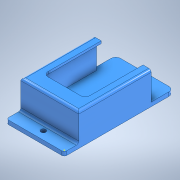
# Autodesk Inventor part: Camera_Mount
Saved by Autodesk Inventor 2022 (Build 260153000, 153)
## iProperties
Created: 2021-06-15
Part Number: Camera_Mount
Material: Generic
Document SubType Name: Modeling
Designer: Jorian Brusind
Density: 1 g/cm^3
Appearance: Cyan
Author: Jorian Brusind
Autodesk Inventor part; units mm, degrees
ref_plane "YZ Plane" through (0, 0, 0) normal (1, 0, 0) x (0, 1, 0)
ref_plane "XZ Plane" through (0, 0, 0) normal (0, 1, 0) x (-1, 0, 0)
ref_plane "XY Plane" through (0, 0, 0) normal (0, 0, 1) x (1, 0, 0)
sketch "Sketch1" plane through (0, 0, 0) normal (0, 1, 0) x (-1, 0, 0)
  line L0 (0, 0) -> (68, 0)
  line L1 (68, 0) -> (68, -132)
  line L2 (68, -132) -> (0, -132)
  line L3 (0, -132) -> (0, 0)
  line L4 (70, -134) -> (70, 2)
  line L5 (70, 2) -> (-2, 2)
  line L6 (-2, 2) -> (-2, -134)
  line L7 (-2, -134) -> (70, -134)
  dimension "d0" = 68
  dimension "d1" = 132
  dimension "d2" = 2
  constraints: 16 end point, 4 parallel, 2 perpendicular, 1 horizontal, 3 other
  measures "d0" distance of L1.end L2.end
  measures "d1" distance of L0.end L1.end
  measures "d2" distance between parallel lines of L1 L4
extrude "Extrusion1" add sketch "Sketch1" along normal blind 3 contours L0 L1 L2 L3 | L7 L6 L5 L4
sketch "Sketch2" plane through (0, 3, 0) normal (0, 1, 0) x (1, 0, 0)
  line L0 (2, 134) -> (-70, 134) projected
  line L1 (-70, -2) -> (2, -2) projected
  line L2 (-70, 134) -> (2, 134)
  line L3 (2, 134) -> (2, -2)
  line L4 (2, -2) -> (-70, -2)
  line L5 (-70, -2) -> (-70, 134)
  line L6 (-70, 134) -> (-70, -2) projected
  line L7 (-70, 66) -> (2, 66)
  line L8 (2, -2) -> (2, 134) projected
  line L9 (-2, 106) -> (-66, 106)
  line L10 (-66, 106) -> (-66, 20)
  line L11 (-66, 20) -> (-2, 20)
  line L12 (-2, 20) -> (-2, 106)
  line L13 (2, 110) -> (-70, 110)
  line L14 (-70, 110) -> (-70, 16)
  line L15 (-70, 16) -> (2, 16)
  line L16 (2, 16) -> (2, 110)
  line L17 (-66, 106) -> (-70, 106)
  line L18 (-2, 106) -> (2, 106)
  point P0 (0, 0)
  point P1 (-70, -2)
  point P2 (-34, 66)
  point P3 (-30, 72)
  point P4 (-70, 106)
  point P5 (-70, 16)
  point P6 (2, 16)
  point P7 (2, 106)
  dimension "d113" = 64
  dimension "d114" = 86
  dimension "d115" = 72
  dimension "d116" = 94
  dimension "d149" = 40
  dimension "d150" = 44
  dimension "d180" = 32
  dimension "d181" = 36
  constraints: 30 end point, 6 parallel, 4 perpendicular, 3 horizontal, 3 midpoint, 3 point on line
  measures "d113" distance of L11.end L10.end
  measures "d114" distance of L10.end L9.end
  measures "d115" distance of L15.end L14.end
  measures "d116" distance of L14.end L13.end
  measures "d149" distance between parallel lines of L9 L7
  measures "d150" distance between parallel lines of L13 L7
  measures "d180" distance from line of point (-34, 66) L10
  measures "d181" distance from line of L14 point (-34, 66)
extrude "Extrusion2" add sketch "Sketch2" along normal blind 32 contours L3 L7 L12 L18 | L17 L10 L7 L5 | L3 L15 L5 L7 L10 L11 L12
sketch "Sketch3" plane through (0, 0, 0) normal (0, -1, 0) x (1, 0, 0)
  circle A0 centre (-34, -96) radius 2
  circle A1 centre (-34, -36) radius 2
  circle A2 centre (-51.5, -66) radius 2
  circle A3 centre (-16.5, -66) radius 2
  line L0 (2, -134) -> (-70, -134) projected
  line L1 (-70, -134) -> (-70, 2) projected
  line L2 (-70, -66) -> (2, -66)
  line L3 (2, 2) -> (2, -134) projected
  point P0 (0, 0)
  dimension "d10" = 4
  dimension "d13" = 60
  dimension "d14" = 35
  dimension "d15" = 17.5
  dimension "d16" = 30
  dimension "d17" = 30
  dimension "d18" = 17.5
  dimension "d117" = 30
  dimension "d202" = 36
  constraints: 4 centre point, 3 equal radius, 2 end point, 2 midpoint
  measures "d10" diameter of A1
  measures "d13" distance of A1.centre A0.centre
  measures "d14" distance of A3.centre A2.centre
  measures "d15" horizontal distance of A2.centre A0.centre
  measures "d16" vertical distance of A3.centre A0.centre
  measures "d17" vertical distance of A0.centre A2.centre
  measures "d18" horizontal distance of A1.centre A3.centre
  measures "d117" distance from line of L2 A0.centre
  measures "d202" distance from line of L1 A0.centre
extrude "Extrusion3" cut sketch "Sketch3" against normal through all contours A0 | A1 | L2 A2 | A2 L2 | L2 A3 | A3 L2
ref_plane "Work Plane3" through (-62, 3, 10) normal (0, 1, 0) x (1, 0, 0)
ref_plane "Work Plane4" through (-62, 30, 10) normal (0, 1, 0) x (1, 0, 0)
move faces "Move2" translate (0, -2, 0) faces at (-34.0804, 0, -10.0049)
fillet "Fillet17" radius 6 2 edges at (-70, 0.5, -134) (2, 0.5, -134)
ref_plane "Work Plane5" through (-9, -2, 2) normal (0, -1, 0) x (1, 0, 0)
ref_plane "Work Plane7" through (-62, 35, 10) normal (0, 1, 0) x (1, 0, 0)
ref_plane "Work Plane6" through (-62, 35, 10) normal (0, 1, 0) x (1, 0, 0)
sketch "Sketch16" plane through (0, 3, 0) normal (0, 1, 0) x (1, 0, 0)
  line L0 (-2, -2) -> (-66, -2) projected
  line L1 (-34, -2) -> (-34, 8)
  line L2 (-4, 134) -> (-64, 134) projected
  line L3 (-34, 134) -> (-34, 124)
  line L4 (-34, 134) -> (-24, 134) construction
  circle A0 centre (-34, 8) radius 3
  circle A1 centre (-34, 124) radius 3
  point P0 (0, 0)
  point P1 (2, -2)
  point P2 (-70, -2)
  dimension "d164" = 10
  dimension "d165" = 10
  dimension "d166" = 90
  dimension "d167" = 6
  dimension "d168" = 6
  constraints: 6 end point, 2 centre point, 2 coincident, 2 midpoint, 2 vertical, 1 horizontal, 1 perpendicular
  measures "d164" distance of L1.start L1.end
  measures "d165" distance of L3.start L3.end
  measures "d166" angle of L3 L4
  measures "d167" diameter of A0
  measures "d168" diameter of A1
extrude "Extrusion18" cut sketch "Sketch16" against normal through all
sketch "Sketch17" plane through (0, 35, 0) normal (0, 1, 0) x (1, 0, 0)
  line L0 (2, 16) -> (-70, 16) projected
  line L1 (-2, 16) -> (-66, 16)
  line L2 (-66, 16) -> (-66, 34)
  line L3 (-66, 34) -> (-2, 34)
  line L4 (-2, 34) -> (-2, 16)
  line L5 (-70, 106) -> (-60, 106)
  line L6 (-60, 106) -> (-60, 16)
  line L7 (-60, 16) -> (-70, 16)
  line L8 (-70, 16) -> (-70, 106)
  line L9 (2, 16) -> (2, 106) projected
  line L10 (2, 106) -> (-8, 106)
  line L11 (-8, 106) -> (-8, 16)
  line L12 (-8, 16) -> (2, 16)
  line L13 (2, 16) -> (2, 106)
  point P0 (-66, 16)
  point P1 (2, 34)
  point P2 (-60, 16)
  point P3 (-8, 16)
  point P4 (2, 34)
  point P5 (-8, 34)
  point P6 (-60, 34)
  dimension "d190" = 10
  dimension "d191" = 90
  dimension "d192" = 10
  dimension "d193" = 90
  constraints: 24 end point, 6 parallel, 3 horizontal, 3 perpendicular
  measures "d190" distance of L6.end L0.end
  measures "d191" distance of L5.end L6.end
  measures "d192" distance of L0.start L11.end
  measures "d193" distance of L11.end L10.end
extrude "Extrusion19" add sketch "Sketch17" along normal blind 3
fillet "Fillet32" radius 6 2 edges at (-8, 36.5, -34) (-60, 36.5, -34)
fillet "Fillet33" radius 3 5 edges at (-66, 35, -63) (-2, 35, -63) (-34, 38, -16) (2, 38, -61) (-70, 38, -61)
fillet "Fillet34" radius 3 1 edges at (-34, 3, -16)
fillet "Fillet36" radius 3 2 edges at (-70, 0.5, 2) (2, 0.5, 2)
fillet "Fillet37" radius 3 1 edges at (-34, 35, -20)
sketch "Sketch18" plane through (0, 3, 0) normal (0, 1, 0) x (1, 0, 0)
  point P0 (0, 0)
body "Solid1"
